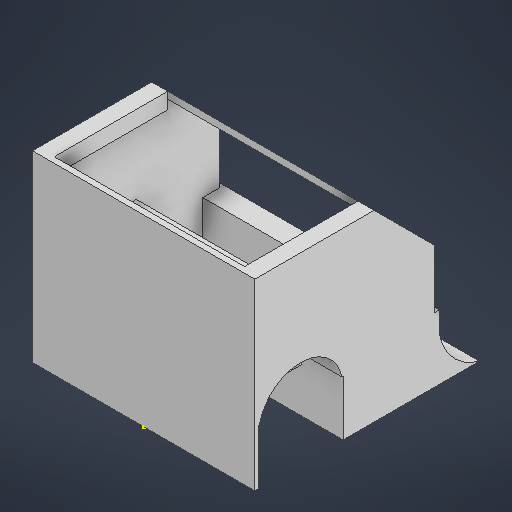
# Autodesk Inventor part: Mini Sumô Definitivo - CHASSI
Saved by Autodesk Inventor 2026.1 (Build 301233000, 233)
## iProperties
Created: 2025-12-03
Part Number: Mini Sumô Definitivo - CHASSI
Material: Genérico
Document SubType Name: Modeling
Designer: panto
Density: 1 g/cm^3
Appearance: Padrão
Author: panto
Autodesk Inventor part; units mm, degrees
ref_plane "YZ Plane" through (0, 0, 0) normal (1, 0, 0) x (0, 1, 0)
ref_plane "XZ Plane" through (0, 0, 0) normal (0, 1, 0) x (-1, 0, 0)
ref_plane "XY Plane" through (0, 0, 0) normal (0, 0, 1) x (1, 0, 0)
sketch "Esboço1" plane through (0, 0, 0) normal (1, 0, 0) x (0, 1, 0)
  line L0 (0, 0) -> (80, 0)
  line L1 (80, 0) -> (80, -52)
  line L2 (80, -97) -> (0, -97)
  line L3 (0, -97) -> (0, 0)
  line L4 (80, 0) -> (0, 0)
  line L5 (0, 0) -> (0, -60)
  line L6 (80, -60) -> (80, 0)
  line L7 (0, 0) -> (0, -19.5)
  line L8 (19.5, 0) -> (0, 0)
  line L9 (0, -98) -> (0, -97)
  line L10 (0, -97) -> (40, -97)
  line L11 (0, 0) -> (0, -20)
  line L12 (80, 0) -> (80, -52)
  line L13 (80, -52) -> (0, -52)
  line L14 (0, -52) -> (0, -97)
  line L15 (0, -97) -> (80, -97)
  line L16 (80, -97) -> (80, -52)
  line L17 (0, -74.5) -> (0, -97)
  line L18 (0, -97) -> (80, -97)
  line L19 (80, -97) -> (80, -74.5)
  line L20 (80, -52) -> (80, -78.5)
  line L21 (53.5, -78.5) -> (28.1691, -78.5)
  line L22 (80, -52) -> (53.5, -78.5)
  arc A0 (0.0257, -97) -> (0, -98) centre (19.5, -98) ccw
  line L23 (80, -52) -> (80, -54)
  line L24 (80, -54) -> (53.5, -80.533)
  line L25 (53.5, -80.533) -> (28.1691, -80.533)
  line L26 (28.1691, -80.533) -> (28.1691, -78.5)
  arc A1 (18.9926, -80.533) -> (0, -98) centre (23.5809, -104.5813) ccw
  line L27 (28.1691, -80.533) -> (18.9926, -80.533)
  circle A2 centre (20, -20) radius 18.5
  line L28 (20, -38.5) -> (0, -38.5)
  line L29 (20, -1.5) -> (0, -1.5)
  point P0 (0, -78.5)
  point P1 (80, -78.5)
  point P2 (0.3022, -97)
  dimension "d0" = 80
  dimension "d1" = 97
  dimension "d6" = 20
  dimension "d13" = 52
  dimension "d14" = 26.5
  dimension "d15" = 26.5
  dimension "d16" = 26.5
  dimension "d17" = 19.5
  dimension "d19" = 2
  dimension "d20" = 37.5
  dimension "d75" = 37
  constraints: 60 end point, 16 point on line, 8 perpendicular, 6 parallel, 6 point on circle, 4 tangent, 3 centre point, 3 horizontal, 1 collinear, 1 midpoint
  measures "d0" distance of L2.start L2.end
  measures "d1" distance of L2.end L0.start
  measures "d6" distance of L4.end L11.end
  measures "d13" distance of L0.end L12.end
  measures "d14" distance of L12.end L20.end
  measures "d15" distance of L1.end point (80, -78.5)
  measures "d16" distance of L21.start point (80, -78.5)
  measures "d17" radius of A0
  measures "d19" distance of L1.end L23.end
  measures "d20" distance of L23.end L24.end
  measures "d75" diameter of A2
sketch "Esboço2" plane through (0, 0, 0) normal (1, 0, 0) x (0, 1, 0)
  point P0 (0, 0)
extrude "Extrusão1" add sketch "Esboço1" along normal mid plane 97 contours L0 L1 L13 L3 L28 A2 L29 | L29 A2 L28 L3 | A2 | L22 L21 L26 L27 A1 L2 L3 L13 | L2 A0 L9 | A1 A0 L2
sketch "Esboço3" plane through (0, 0, 0) normal (1, 0, 0) x (0, 1, 0)
  line L0 (0, 0) -> (80, 0) projected
  line L1 (80, 0) -> (80, -2.5)
  line L2 (80, 0) -> (80, -52) projected
  line L3 (80, -2.5) -> (80, -5)
  line L4 (80, -2.5) -> (77, -2.5)
  line L5 (53.5, -78.5) -> (28.1691, -78.5) projected
  line L6 (77, -2.5) -> (42, -2.5)
  line L7 (42, -2.5) -> (42, -78.5)
  line L8 (42, -78.5) -> (77, -78.5)
  line L9 (77, -78.5) -> (77, -2.5)
  line L10 (28.1691, -78.5) -> (31.1691, -78.5)
  line L11 (28.1691, -78.5) -> (42, -78.5)
  line L12 (42, -78.5) -> (42, -40.5)
  line L13 (28.1691, -78.5) -> (42, -78.5)
  line L14 (42, -78.5) -> (42, -42.2949)
  line L15 (42, -42.2949) -> (28.1691, -42.2949)
  line L16 (28.1691, -42.2949) -> (28.1691, -78.5)
  line L17 (28.1691, -42.2949) -> (4.792, -42.2949)
  line L18 (4.792, -42.2949) -> (4.792, -71.2859)
  line L19 (4.792, -71.2859) -> (28.1691, -71.2859)
  point P0 (20, 0)
  dimension "d27" = 2.5
  dimension "d28" = 2.5
  dimension "d29" = 3
  dimension "d30" = 35
  constraints: 34 end point, 6 point on line, 4 parallel, 4 perpendicular, 3 horizontal, 1 midpoint, 1 vertical
  measures "d27" distance of L0.end L1.end
  measures "d28" distance of L1.end L3.end
  measures "d29" distance of L1.end L4.end
  measures "d30" distance of L8.end L7.end
extrude "Extrusão2" cut sketch "Esboço3" along normal mid plane 91
sketch "Esboço4" plane through (-48.5, 80, 0) normal (0, 1, 0) x (1, 0, 0)
  line L0 (0, 0) -> (0, 52) projected
  line L1 (0, 0) -> (97, 0) projected
  line L2 (3, 2.5) -> (3, 55) projected
  line L3 (94, 2.5) -> (3, 2.5) projected
  line L4 (3, 2.5) -> (93.6926, 2.5)
  line L5 (93.6926, 2.5) -> (93.6926, 52)
  line L6 (93.6926, 52) -> (3, 52)
  line L7 (3, 52) -> (3, 2.5)
  point P0 (48.5, 0)
  constraints: 8 end point, 2 parallel, 1 horizontal, 1 perpendicular
extrude "Extrusão3" cut sketch "Esboço4" against normal blind 8.5
sketch "Esboço5" plane through (-45.5, 77, -52) normal (0, 0, 1) x (1, 0, 0)
  line L0 (91, 0) -> (0, 0) projected
  line L1 (0, 0) -> (4, 0)
  line L2 (4, 0) -> (4, -4)
  line L3 (4, -4) -> (0, -4)
  line L4 (0, -4) -> (0, 0)
  line L5 (91, -23.5) -> (91, 0) projected
  line L6 (91, 0) -> (87, 0)
  line L7 (87, 0) -> (87, -4)
  line L8 (87, -4) -> (91, -4)
  line L9 (91, -4) -> (91, 0)
  line L10 (0, 3) -> (0, 0) projected
  line L11 (0, 3) -> (4, 3)
  line L12 (4, 3) -> (4, 0)
  line L13 (4, 0) -> (0, 0)
  line L14 (0, 0) -> (0, 3)
  line L15 (87, 3) -> (91, 3)
  line L16 (91, 3) -> (91, 0)
  line L17 (91, 0) -> (87, 0)
  line L18 (87, 0) -> (87, 3)
  point P0 (45.5, -77)
  point P1 (91, -4)
  dimension "d38" = 4
  dimension "d39" = 4
  dimension "d40" = 4
  constraints: 32 end point, 8 parallel, 4 horizontal, 4 perpendicular
  measures "d38" distance of L2.end L3.end
  measures "d39" distance of L1.end L2.end
  measures "d40" distance of L8.end L7.end
extrude "Extrusão4" add sketch "Esboço5" along normal blind 49.5
sketch "Esboço6" plane through (45.5, 4.792, -42.2949) normal (0, 0, -1) x (-1, 0, 0)
  line L0 (0, 37.208) -> (0, 33.208)
  line L1 (17, 33.208) -> (27, 33.208)
  line L2 (27, 33.208) -> (27, 23.208)
  line L3 (27, 23.208) -> (17, 23.208)
  line L4 (17, 23.208) -> (17, 33.208)
  line L5 (0, 37.208) -> (91, 37.208) projected
  line L6 (91, 37.208) -> (87, 37.208)
  line L7 (-3, 35.208) -> (94, 35.208) projected
  line L8 (91, 37.208) -> (91, 33.208)
  line L9 (74, 33.208) -> (64, 33.208)
  line L10 (64, 33.208) -> (64, 23.208)
  line L11 (64, 23.208) -> (74, 23.208)
  line L12 (74, 23.208) -> (74, 33.208)
  line L13 (91, 33.208) -> (74, 33.208)
  point P0 (45.5, -4.792)
  dimension "d43" = 4
  dimension "d44" = 17
  dimension "d45" = 10
  dimension "d46" = 10
  dimension "d52" = 10
  dimension "d53" = 10
  dimension "d54" = 17
  constraints: 24 end point, 4 parallel, 2 horizontal, 2 perpendicular, 2 vertical, 1 collinear, 1 point on line
  measures "d43" distance of L0.start L0.end
  measures "d44" distance of L0.end L1.start
  measures "d45" distance of L2.end L3.end
  measures "d46" distance of L1.end L2.end
  measures "d52" distance of L11.end L10.end
  measures "d53" distance of L10.end L9.end
  measures "d54" distance of L8.end L9.start
extrude "Extrusão5" cut sketch "Esboço6" against normal blind 14 contours L12 L11 L10 L9 | L1 L2 L3 L4
sketch "Esboço9" plane through (48.5, 0, 0) normal (1, 0, 0) x (0, 0, -1)
  circle A0 centre (20, 20) radius 18.5
  line L0 (1.5, 20) -> (1.5, 0)
  line L1 (98, 0) -> (0, 0) projected
  line L2 (38.5, 20) -> (38.5, 0)
  line L3 (20, 24) -> (1.9376, 24)
  line L4 (20, 24) -> (38.0624, 24)
  line L5 (20, 19.5) -> (38.5, 19.5)
  line L6 (20, 19.5) -> (1.5, 19.5)
  point P0 (38.5, 0)
  point P1 (1.5068, 19.5)
  point P2 (38.4932, 19.5)
  dimension "d76" = 37
  dimension "d81" = 4.5
  constraints: 12 end point, 4 point on circle, 4 point on line, 2 vertical, 1 centre point, 1 horizontal, 1 perpendicular
  measures "d76" diameter of A0
  measures "d81" distance of L3.start L5.start
extrude "Extrusão7" cut sketch "Esboço9" against normal blind 97
extrude "Extrusão8" add sketch "Esboço9" against normal blind 97 contours A0 L5 L6 L3 L4
sketch "Esboço10" plane through (48.5, 19.5, -38.4932) normal (0, -1, 0) x (1, 0, 0)
  line L0 (-97, 0) -> (-97, 36.9865) projected
  line L1 (0, -13.5068) -> (0, 38.4932) projected
  line L2 (0, 0.4309) -> (0, 36.5556) projected
  line L3 (0, -0.0068) -> (-97, -0.0068) projected
  line L4 (-97, 36.9865) -> (-79, 36.9865)
  line L5 (-79, 36.9865) -> (-79, -0.0068)
  line L6 (-79, -0.0068) -> (-97, -0.0068)
  line L7 (-97, -0.0068) -> (-97, 36.9865)
  line L8 (0, 36.9865) -> (-97, 36.9865) projected
  line L9 (-18, 36.9865) -> (0, 36.9865)
  line L10 (0, 36.9865) -> (0, -0.0068)
  line L11 (0, -0.0068) -> (-18, -0.0068)
  line L12 (-18, -0.0068) -> (-18, 36.9865)
  point P0 (-48.5, 38.4932)
  constraints: 16 end point, 4 parallel, 2 horizontal, 2 perpendicular, 2 point on line
extrude "Extrusão9" cut sketch "Esboço10" against normal blind 4.5 contours L0 L4 L5 L3 L7 | L8 L1 L3 L12
sketch "Esboço11" plane through (-30.5, 19.5, -1.5068) normal (0, -1, 0) x (1, 0, 0)
  line L0 (0, 0) -> (0, -36.9865) projected
  line L1 (0, -36.9865) -> (0, -28.7365)
  line L2 (-18, 0) -> (0, 0) projected
  line L3 (0, 0) -> (0, -8.25)
  line L4 (0, -28.7365) -> (0, -8.25)
  line L5 (61, 0) -> (61, -8.25)
  line L6 (61, -36.9865) -> (61, 0) projected
  line L7 (61, -36.9865) -> (61, -28.7365)
  line L8 (61, -28.7365) -> (61, -8.25)
  line L9 (61, -18.4932) -> (33, -18.4932)
  line L10 (33, -18.4932) -> (37, -18.4932)
  line L11 (61, -18.4932) -> (57, -18.4932)
  line L12 (37, -8.25) -> (47, -8.25)
  line L13 (47, -8.25) -> (47, -28.7365)
  line L14 (47, -28.7365) -> (37, -28.7365)
  line L15 (37, -28.7365) -> (37, -8.25)
  line L16 (38, -18.4932) -> (34, -18.4932)
  line L17 (24, -8.25) -> (14, -8.25)
  line L18 (14, -8.25) -> (14, -28.7365)
  line L19 (14, -28.7365) -> (24, -28.7365)
  line L20 (24, -28.7365) -> (24, -8.25)
  line L21 (24, -18.4932) -> (28, -18.4932)
  line L22 (24, -18.4932) -> (0, -18.4932)
  line L23 (28, -8.25) -> (33, -8.25)
  line L24 (33, -8.25) -> (33, -3.25)
  line L25 (33, -3.25) -> (28, -3.25)
  line L26 (28, -3.25) -> (28, -8.25)
  line L27 (28, -28.7365) -> (33, -28.7365)
  line L28 (33, -28.7365) -> (33, -33.7365)
  line L29 (33, -33.7365) -> (28, -33.7365)
  line L30 (28, -33.7365) -> (28, -28.7365)
  point P0 (30.5, 1.5068)
  dimension "d91" = 8.25
  dimension "d92" = 8.25
  dimension "d96" = 28
  dimension "d100" = 4
  dimension "d101" = 4
  dimension "d102" = 4
  dimension "d105" = 5
  dimension "d106" = 5
  dimension "d107" = 5
  dimension "d108" = 5
  constraints: 56 end point, 8 parallel, 7 point on line, 5 horizontal, 4 perpendicular, 2 midpoint
  measures "d91" distance of L0.end L1.end
  measures "d92" distance of L0.start L3.end
  measures "d96" distance of L9.start L9.end
  measures "d100" distance of L9.end L10.end
  measures "d101" distance of L9.start L11.end
  measures "d102" distance of L16.start L16.end
  measures "d105" distance of L25.end L24.end
  measures "d106" distance of L24.end L23.end
  measures "d107" distance of L28.end L29.end
  measures "d108" distance of L27.end L28.end
extrude "Extrusão10" cut sketch "Esboço11" against normal blind 4.5 contours L26 L25 L24 L23 | L27 L28 L29 L30
equation "\"d16\" = d15"
